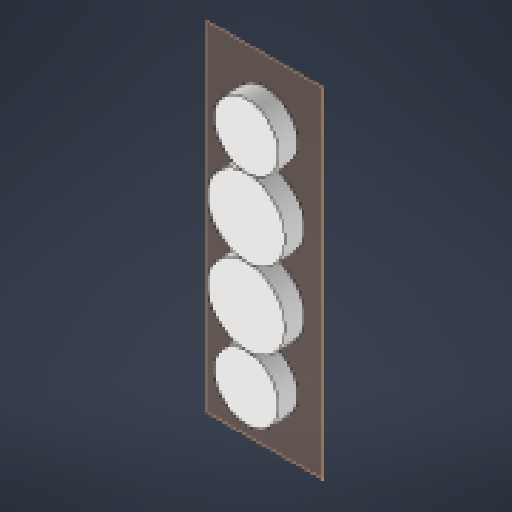
# Autodesk Inventor part: gearTemplate
Saved by Autodesk Inventor 2024.3 (Build 283343000, 343)
## iProperties
Created: 2025-03-10
Part Number: gearTemplate
Material: Generic
Document SubType Name: Modeling
Designer: jings
Density: 1 g/cm^3
Appearance: Default
Author: jings
Autodesk Inventor part; units mm, degrees
ref_plane "YZ Plane" through (0, 0, 0) normal (1, 0, 0) x (0, 1, 0)
ref_plane "XZ Plane" through (0, 0, 0) normal (0, 1, 0) x (-1, 0, 0)
ref_plane "XY Plane" through (0, 0, 0) normal (0, 0, 1) x (1, 0, 0)
ref_plane "Work Plane1" through (0, 0, 0) normal (0, 0, 1) x (1, 0, 0)
sketch "Sketch1" plane through (0, 0, 0) normal (0, 0, 1) x (1, 0, 0)
  circle A0 centre (0, -107.5508) radius 31.75 projected
  circle A1 centre (0, 108.3492) radius 31.75 projected
  circle A2 centre (0, 38.4992) radius 38.1 projected
  circle A3 centre (0, -37.7008) radius 38.1 projected
  point P0 (0, 0)
  point P1 (0, -75.8008)
  point P2 (0, 0.3992)
  point P3 (0, 76.5992)
extrude "Extrusion1" add sketch "Sketch1" along normal blind 19.05
body "Solid1"
